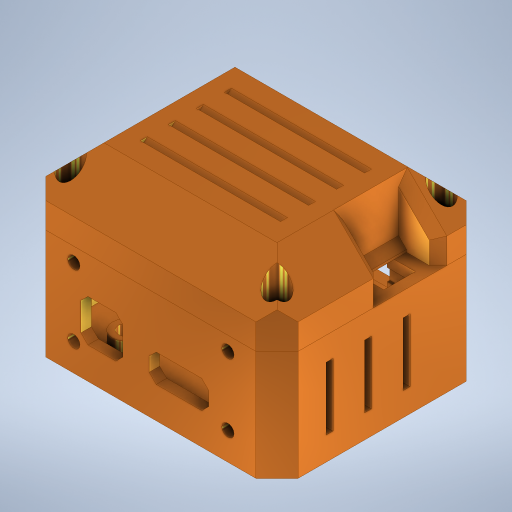
# Autodesk Inventor part: ModuloIndBase
Saved by Autodesk Inventor 2024.2 (Build 282272000, 272)
## iProperties
Created: 2024-09-07
Part Number: ModuloIndBase
Material: Generic
Document SubType Name: Modeling
Designer: Admin
Density: 1 g/cm^3
Appearance: Metal 1600F Hot
Author: Admin
Autodesk Inventor part; units mm, degrees
ref_plane "YZ Plane" through (0, 0, 0) normal (1, 0, 0) x (0, 1, 0)
ref_plane "XZ Plane" through (0, 0, 0) normal (0, 1, 0) x (-1, 0, 0)
ref_plane "XY Plane" through (0, 0, 0) normal (0, 0, 1) x (1, 0, 0)
sketch "Sketch1" plane through (0, 0, 0) normal (0, 1, 0) x (-1, 0, 0)
  line L0 (30, 36) -> (-30, 36)
  line L1 (-30, 36) -> (-30, -36)
  line L2 (-30, -36) -> (30, -36)
  line L3 (30, -36) -> (30, 36)
  line L4 (30, 36) -> (-30, -36) construction
  line L5 (-30, 36) -> (30, -36) construction
  point P0 (0, 0)
  dimension "d0" = 72
  dimension "d1" = 60
  constraints: 12 end point, 2 midpoint, 2 parallel, 1 horizontal, 1 perpendicular
  measures "d0" distance of L2.end L0.start
  measures "d1" distance of L0.start L0.end
extrude "BaseBlock" add sketch "Sketch1" along normal blind 50
chamfer "ExteriorDetail" distance 6 angle 45 4 edges at (-30, 25, 36) (30, 25, 36) (30, 25, -36) (-30, 25, -36)
chamfer "ExteriorShell" distance 11.3 angle 45 4 edges at (-30, 0, 0) (0, 0, 36) (30, 0, 0) (0, 0, -36)
shell "Shell1" thickness 3 removed faces 1 at (10, 50, -10)
ref_plane "Work Plane1" through (0, 18.6, 0) normal (0, 1, 0) x (1, 0, 0)
split body "Split1" result two bodies by plane through (0, 18.6, 0) normal (0, 1, 0) first body at (29.5, 29.0667, 10)
sketch "Sketch2" plane through (0, 50, 0) normal (0, 1, 0) x (1, 0, 0)
  line L0 (30, -30) -> (30, 30) projected
  line L1 (24, 36) -> (30, 30) projected
  line L2 (-27, 28.7574) -> (-22.7574, 33) projected
  line L3 (-22.7574, 33) -> (22.7574, 33) projected
  line L4 (22.7574, 33) -> (27, 28.7574) projected
  line L5 (27, 28.7574) -> (27, -28.7574) projected
  line L6 (27, -28.7574) -> (22.7574, -33) projected
  line L7 (22.7574, -33) -> (-22.7574, -33) projected
  line L8 (-22.7574, -33) -> (-27, -28.7574) projected
  line L9 (-27, -28.7574) -> (-27, 28.7574) projected
  line L10 (-30, 30) -> (-24, 36) projected
  line L11 (-30, 30) -> (-30, -30) projected
  line L12 (-24, -36) -> (-30, -30) projected
  line L13 (-24, -36) -> (24, -36) projected
  line L14 (30, -30) -> (24, -36) projected
  line L15 (30, -30) -> (30, 30) projected
  line L16 (24, 36) -> (30, 30) projected
  line L17 (24, 36) -> (-24, 36) projected
  point P0 (0, 0)
extrude "Extrusion2" add sketch "Sketch2" against normal blind 3 contours L14 L13 L12 L11 L10 L17 L1 L0 | L2 L3 L4 L5 L6 L7 L8 L9 bodies 2
sketch "Sketch4" plane through (-24, 18.6, -36) normal (0, -1, 0) x (1, 0, 0)
  line L0 (46.7574, 69) -> (51, 64.7574) projected
  line L1 (48.8787, 66.8787) -> (47.4645, 65.4645)
  line L2 (48.8787, 66.8787) -> (50.8787, 66.8787) construction
  circle A0 centre (47.4645, 65.4645) radius 2.25
  circle A1 centre (47.4645, 65.4645) radius 4
  line L3 (51, 64.7574) -> (51, 7.2426) projected
  line L4 (51, 36) -> (-3, 36) construction
  line L5 (-3, 7.2426) -> (-3, 64.7574) projected
  line L6 (51, 36) -> (105, 36) construction
  line L7 (24, 36) -> (24, 26) construction
  circle A2 centre (47.4645, 6.5355) radius 2.25
  circle A3 centre (47.4645, 6.5355) radius 4
  circle A4 centre (0.5355, 65.4645) radius 2.25
  circle A5 centre (0.5355, 65.4645) radius 4
  circle A6 centre (0.5355, 6.5355) radius 2.25
  circle A7 centre (0.5355, 6.5355) radius 4
  point P0 (48.1498, 67.6075)
  point P1 (49.6075, 66.1498)
  dimension "d23" = 2
  dimension "d24" = 135
  dimension "d25" = 4.5
  dimension "d27" = 8
  constraints: 10 end point, 8 centre point, 6 symmetric about line, 5 coincident, 4 midpoint, 2 equal length, 2 horizontal, 1 perpendicular, 1 vertical, 6 other
  measures "d23" distance of L1.start L1.end
  measures "d24" angle of L1 L2
  measures "d25" diameter of A0
  measures "d27" diameter of A1
extrude "Extrusion3" add sketch "Sketch4" against normal through all bodies 2
extrude "Extrusion4" cut sketch "Sketch4" against normal through all contours A0 L0 | L0 A0 | A2 | A4 | A6 bodies 2
sketch "Sketch5" plane through (0, 47, 0) normal (0, -1, 0) x (1, 0, 0)
  line L0 (0, 0) -> (1, 0) construction
  line L1 (-18, -19) -> (20, -19) construction
  line L2 (20, -19) -> (20, 19) construction
  line L3 (20, 19) -> (-18, 19) construction
  line L4 (-18, 19) -> (-18, -19) construction
  line L5 (-18, -19) -> (20, 19) construction
  line L6 (20, -19) -> (-18, 19) construction
  circle A0 centre (-18, -19) radius 1.6
  line L7 (-30, 30) -> (-30, -30) projected
  circle A1 centre (-18, -19) radius 4
  circle A2 centre (-18, -19) radius 2.275
  circle A3 centre (20, -19) radius 4
  circle A4 centre (20, -19) radius 2.275
  circle A5 centre (20, -19) radius 1.6
  circle A6 centre (20, 19) radius 4
  circle A7 centre (20, 19) radius 2.275
  circle A8 centre (20, 19) radius 1.6
  circle A9 centre (-18, 19) radius 4
  circle A10 centre (-18, 19) radius 2.275
  circle A11 centre (-18, 19) radius 1.6
  circle A12 centre (20, 19) radius 3.5
  dimension "d35" = 38
  dimension "d36" = 38
  dimension "d38" = 12
  dimension "d39" = 3.2
  dimension "d40" = 8
  dimension "d41" = 4.55
  dimension "d44" = 360
  dimension "d50" = 7
  constraints: 14 end point, 13 centre point, 7 coincident, 2 horizontal, 2 midpoint, 2 parallel, 1 perpendicular, 25 other
  measures "d35" distance of L3.end L2.end
  measures "d36" distance of L2.end L1.end
  measures "d38" distance between parallel lines of L4 L7
  measures "d39" diameter of A0
  measures "d40" diameter of A1
  measures "d41" diameter of A2
  measures "d50" diameter of A12
extrude "Extrusion5" cut sketch "Sketch5" against normal blind 3.2 contours A0 | A5 | A7 | A8 | A11 bodies 2
extrude "Extrusion6" add sketch "Sketch5" along normal blind 3.2 contours A1 | A3 | A9 bodies 2
extrude "Extrusion7" add sketch "Sketch5" along normal blind 3.2 contours A12 bodies 2
sketch "Sketch6" plane through (-21.5936, 47, -33) normal (0, 0, 1) x (1, 0, 0)
  line L0 (43.1873, 0) -> (0, 0) projected
  line L1 (-2.4064, -28.4) -> (45.5936, -28.4) projected
  line L2 (29.5936, 0) -> (21.5936, 0)
  line L3 (21.5936, 0) -> (21.5936, -28.4)
  line L4 (21.5936, -28.4) -> (29.5936, -28.4)
  line L5 (29.5936, -28.4) -> (29.5936, 0)
  line L6 (-8.4064, -28.4) -> (-8.4064, 3) projected
  line L7 (29.5936, -28.4) -> (25.0936, -28.4)
  line L8 (25.0936, -28.4) -> (25.0936, -25.4)
  line L9 (25.0936, -25.4) -> (29.5936, -25.4)
  line L10 (29.5936, -25.4) -> (29.5936, -28.4)
  line L11 (29.5936, -25.4) -> (24.3936, -25.4)
  line L12 (24.3936, -25.4) -> (24.3936, -21.9)
  line L13 (24.3936, -21.9) -> (29.5936, -21.9)
  line L14 (29.5936, -21.9) -> (29.5936, -25.4)
  line L15 (29.5936, -21.9) -> (25.0936, -21.9)
  line L16 (25.0936, -21.9) -> (25.0936, -18.9)
  line L17 (25.0936, -18.9) -> (29.5936, -18.9)
  line L18 (29.5936, -18.9) -> (29.5936, -21.9)
  line L19 (29.5936, -18.9) -> (23.5936, -18.9)
  line L20 (23.5936, -18.9) -> (23.5936, 0)
  line L21 (23.5936, 0) -> (29.5936, 0)
  line L22 (29.5936, 0) -> (29.5936, -18.9)
  line L23 (29.5936, 0) -> (37.5936, 0)
  line L24 (37.5936, 0) -> (37.5936, -28.4)
  line L25 (37.5936, -28.4) -> (29.5936, -28.4)
  line L26 (29.5936, -28.4) -> (34.0936, -28.4)
  line L27 (34.0936, -28.4) -> (34.0936, -25.4)
  line L28 (34.0936, -25.4) -> (29.5936, -25.4)
  line L29 (29.5936, -25.4) -> (34.7936, -25.4)
  line L30 (34.7936, -25.4) -> (34.7936, -21.9)
  line L31 (34.7936, -21.9) -> (29.5936, -21.9)
  line L32 (29.5936, -21.9) -> (34.0936, -21.9)
  line L33 (34.0936, -21.9) -> (34.0936, -18.9)
  line L34 (34.0936, -18.9) -> (29.5936, -18.9)
  line L35 (29.5936, -18.9) -> (35.5936, -18.9)
  line L36 (35.5936, -18.9) -> (35.5936, 0)
  line L37 (35.5936, 0) -> (29.5936, 0)
  point P0 (21.5936, -47)
  point P1 (25.0936, -21.9)
  point P2 (23.5936, 0)
  point P3 (21.5936, 0)
  point P4 (34.0936, -28.4)
  point P5 (37.5936, -28.4)
  point P6 (37.5936, 0)
  point P7 (35.5936, 0)
  point P8 (34.0936, -21.9)
  dimension "d53" = 30
  dimension "d54" = 8
  dimension "d55" = 4.5
  dimension "d56" = 3
  dimension "d57" = 3.5
  dimension "d58" = 5.2
  dimension "d59" = 3
  dimension "d60" = 4.5
  dimension "d61" = 2
  constraints: 70 end point, 10 parallel, 10 symmetric about line, 5 horizontal, 5 perpendicular, 3 point on line, 1 midpoint
  measures "d53" distance between parallel lines of L6 L3
  measures "d54" distance between parallel lines of L3 L5
  measures "d55" distance of L8.end L9.end
  measures "d56" distance of L7.end L8.end
  measures "d57" distance of L11.end L12.end
  measures "d58" distance of L12.end L13.end
  measures "d59" distance of L15.end L16.end
  measures "d60" distance of L16.end L17.end
  measures "d61" distance between parallel lines of L3 L20
extrude "Extrusion8" add sketch "Sketch6" along normal blind 8 contours L24 L1 L27 L29 L30 L31 L33 L35 L36 L0 | L20 L19 L16 L13 L12 L11 L8 L1 L3 L0 bodies 2
mirror "Mirror1" about plane through (0, 0, 0) normal (0, 0, 1) of "Extrusion8" bodies 2
sketch "Sketch7" plane through (30, 50, 30) normal (1, 0, 0) x (0, 0, -1)
  line L0 (46.5, -9) -> (29.5, -9)
  line L1 (29.5, -9) -> (29.5, -17)
  line L2 (29.5, -17) -> (46.5, -17)
  line L3 (46.5, -17) -> (46.5, -9)
  line L4 (66, -31.4) -> (66, 0) projected
  line L5 (0, 0) -> (60, 0) projected
  line L6 (22, -21) -> (10, -21)
  line L7 (10, -21) -> (10, -9)
  line L8 (10, -9) -> (22, -9)
  line L9 (22, -9) -> (22, -21)
  line L10 (60, -31.4) -> (0, -31.4) projected
  line L11 (-6, 0) -> (-6, -31.4) projected
  point P0 (30, -50)
  dimension "d72" = 17
  dimension "d73" = 8
  dimension "d74" = 19.5
  dimension "d75" = 9
  dimension "d77" = 16
  dimension "d78" = 12
  dimension "d79" = 12
  dimension "d80" = 9
  constraints: 16 end point, 4 parallel, 2 horizontal, 2 perpendicular
  measures "d72" distance of L1.end L2.end
  measures "d73" distance of L2.end L0.start
  measures "d74" distance between parallel lines of L4 L3
  measures "d75" distance between parallel lines of L5 L0
  measures "d77" distance between parallel lines of L11 L7
  measures "d78" distance of L7.end L8.end
  measures "d79" distance of L8.end L6.start
  measures "d80" distance between parallel lines of L5 L8
extrude "Extrusion9" cut sketch "Sketch7" against normal blind 3 bodies 2
mirror "Mirror2" about plane through (0, 0, 0) normal (1, 0, 0) of "Extrusion9" bodies 2
chamfer "Chamfer3" distance 2 angle 45 16 edges at (28.5, 33, -16.5) (28.5, 41, -16.5) (28.5, 41, 0.5) (28.5, 33, 0.5) (28.5, 29, 8) (28.5, 41, 8) (28.5, 41, 20) (28.5, 29, 20) (-28.5, 41, 20) (-28.5, 41, 0.5) (-28.5, 41, 8) (-28.5, 41, -16.5) (-28.5, 33, -16.5) (-28.5, 29, 8) (-28.5, 33, 0.5) (-28.5, 29, 20)
sketch "Sketch9" plane through (30, 50, 30) normal (1, 0, 0) x (0, 0, -1)
  line L0 (60, 0) -> (60, -31.4) construction
  line L1 (60, -31.4) -> (60, -27.4) construction
  line L2 (60, -27.4) -> (52, -27.4) construction
  circle A0 centre (52, -27.4) radius 1.75
  line L3 (2.4064, -31.4) -> (57.5936, -31.4) projected
  line L4 (30, -31.4) -> (30, 0) construction
  line L5 (2.4064, -3) -> (57.5936, -3) projected
  circle A1 centre (8, -27.4) radius 1.75
  circle A2 centre (52, -7.9) radius 1.75
  circle A3 centre (8, -7.9) radius 1.75
  point P0 (30, -50)
  dimension "d87" = 4
  dimension "d88" = 3.5
  dimension "d89" = 8
  dimension "d97" = 19.5
  constraints: 6 end point, 4 centre point, 2 perpendicular, 1 coincident, 1 midpoint, 1 point on line, 1 symmetric about line, 1 vertical, 5 other
  measures "d87" distance of L0.end L1.end
  measures "d88" diameter of A0
  measures "d89" distance of L1.end L2.end
  measures "d97" distance of A0.centre A2.centre
extrude "Extrusion10" cut sketch "Sketch9" against normal blind 3 bodies 2
mirror "Mirror3" about plane through (0, 0, 0) normal (1, 0, 0) of "Extrusion10" bodies 2
sketch "Sketch11" plane through (-24, 50, 36) normal (0, 0, 1) x (1, 0, 0)
  line L0 (10, -24.7) -> (9, -24.7)
  line L1 (9, -24.7) -> (9, -6.7)
  line L2 (9, -6.7) -> (10, -6.7)
  line L3 (10, -6.7) -> (10, -24.7)
  line L4 (48, -31.4) -> (0, -31.4) projected
  line L5 (-6, 0) -> (-6, -31.4) projected
  point P0 (24, -50)
  point P1 (9, -15.7)
  dimension "d108" = 1
  dimension "d109" = 18
  dimension "d110" = 15.7
  dimension "d111" = 15
  constraints: 8 end point, 2 parallel, 1 horizontal, 1 midpoint, 1 perpendicular
  measures "d108" distance of L1.end L2.end
  measures "d109" distance of L0.end L1.end
  measures "d110" distance from line of L4 point (9, -15.7)
  measures "d111" distance between parallel lines of L5 L1
extrude "Extrusion12" cut sketch "Sketch11" against normal through all bodies 2
chamfer "Chamfer4" distance 1 angle 45 4 edges at (-15, 34.3, 36) (-15, 34.3, -36) (-14, 34.3, -33) (-14, 34.3, 33)
pattern_linear "Rectangular Pattern1" count 3 spacing 11 along (1, 0, 0) of "Extrusion12", "Chamfer4" bodies 2
sketch "Sketch14" plane through (-24, 18.6, 36) normal (0, 1, 0) x (1, 0, 0)
  line L0 (51, 3) -> (47.4645, 6.5355) construction
  circle A0 centre (47.4645, 6.5355) radius 4
  circle A1 centre (47.4645, 6.5355) radius 1.6
  line L1 (24, 36) -> (29, 36) construction
  line L2 (24, 36) -> (24, 31) construction
  line L3 (46.7574, 3) -> (51, 7.2426) projected
  circle A2 centre (47.4645, 65.4645) radius 4
  circle A3 centre (47.4645, 65.4645) radius 1.6
  circle A4 centre (0.5355, 6.5355) radius 4
  circle A5 centre (0.5355, 6.5355) radius 1.6
  circle A6 centre (0.5355, 65.4645) radius 4
  circle A7 centre (0.5355, 65.4645) radius 1.6
  dimension "d131" = 8
  dimension "d135" = 90
  constraints: 8 centre point, 6 end point, 6 symmetric about line, 2 coincident, 1 horizontal, 1 vertical, 6 other
  measures "d131" diameter of A0
  measures "d135" angle of L3 L0
extrude "Extrusion14" add sketch "Sketch14" against normal through all bodies 3
sketch "Sketch13" plane through (0, 0, 0) normal (0, -1, 0) x (1, 0, 0)
  line L0 (-27, 33) -> (-23.4645, 29.4645) construction
  line L1 (-27, 33) -> (-22, 33) construction
  circle A0 centre (-23.4645, 29.4645) radius 1.6
  circle A1 centre (-23.4645, 29.4645) radius 3.25
  line L2 (0, 0) -> (-5, 0) construction
  line L3 (0, 0) -> (0, 5) construction
  circle A2 centre (23.4645, 29.4645) radius 1.6
  circle A3 centre (23.4645, 29.4645) radius 3.25
  line L4 (-24, -36) -> (-27, -33)
  line L5 (-27, -33) -> (-23.4645, -29.4645) construction
  line L6 (-27, -33) -> (-22, -33) construction
  circle A4 centre (-23.4645, -29.4645) radius 1.6
  circle A5 centre (-23.4645, -29.4645) radius 3.25
  line L7 (24, -36) -> (-24, -36)
  circle A6 centre (23.4645, -29.4645) radius 1.6
  circle A7 centre (23.4645, -29.4645) radius 3.25
  point P0 (-24, 36)
  point P1 (24, 36)
  dimension "d120" = 5
  dimension "d121" = 45
  dimension "d122" = 3.2
  dimension "d123" = 6.5
  constraints: 16 end point, 11 symmetric about line, 8 centre point, 6 coincident, 2 horizontal, 1 equal length, 1 vertical, 6 other
  measures "d120" distance of L0.start L0.end
  measures "d121" angle of L0 L1
  measures "d122" diameter of A0
  measures "d123" diameter of A1
extrude "Extrusion13" cut sketch "Sketch13" against normal blind 14 contours A0 | A1 | A2 | A3 | A4 | A5 | A6 | A7 bodies 3
sketch "Sketch15" plane through (-24, 18.6, 36) normal (0, 1, 0) x (1, 0, 0)
  line L0 (24, 69) -> (24, 60.7)
  line L1 (24, 60.7) -> (40, 60.7)
  line L2 (40, 60.7) -> (40, 68.7)
  line L3 (54, 66) -> (54, 6) projected
  line L4 (43, 57.7) -> (21, 57.7)
  line L5 (21, 57.7) -> (21, 72)
  line L6 (21, 72) -> (43, 72)
  line L7 (43, 72) -> (43, 57.7)
  line L8 (24, 36) -> (34, 36) construction
  line L9 (40, 60.7) -> (40, 72)
  line L10 (24, 60.7) -> (24, 72)
  line L11 (24, 3) -> (24, 11.3)
  line L12 (24, 11.3) -> (40, 11.3)
  line L13 (40, 11.3) -> (40, 3.3)
  line L14 (43, 14.3) -> (21, 14.3)
  line L15 (21, 14.3) -> (21, 0)
  line L16 (21, 0) -> (43, 0)
  line L17 (43, 0) -> (43, 14.3)
  line L18 (40, 11.3) -> (40, 0)
  line L19 (24, 11.3) -> (24, 0)
  line L20 (0, 72) -> (48, 72) projected
  point P0 (24, 69)
  dimension "d138" = 8
  dimension "d139" = 16
  dimension "d140" = 14
  dimension "d141" = 3
  dimension "d150" = 11.3
  dimension "d151" = 0
  constraints: 38 end point, 10 symmetric about line, 6 point on line, 3 parallel, 2 perpendicular, 1 horizontal, 1 other
  measures "d138" distance of L1.end L2.end
  measures "d139" distance of L0.end L1.end
  measures "d140" distance between parallel lines of L3 L2
  measures "d141" distance between parallel lines of L1 L4
  measures "d150" distance between parallel lines of L6 L1
  measures "d151" distance between parallel lines of L6 L20
extrude "Extrusion15" add sketch "Sketch15" against normal through all contours L0 L1 L2 L9 L6 L7 L4 L5 L10 | L19 L16 L15 L14 L17 L18 L13 L12 L11 bodies 3
extrude "Extrusion16" cut sketch "Sketch15" against normal through all contours L10 L6 L9 L2 L1 L0 | L11 L12 L13 L18 L16 L19 bodies 3
chamfer "Chamfer5" distance 2.5 angle 45 8 edges at (0, 5.65, -30.35) (0, 14.95, -36) (16, 5.65, -30.35) (16, 14.95, -36) (0, 5.65, 30.35) (0, 14.95, 36) (16, 14.95, 36) (16, 5.65, 30.35)
sketch "Sketch17" plane through (0, 0, 0) normal (0, 0, 1) x (1, 0, 0)
  line L0 (0, 0) -> (-11, 0) construction
  line L1 (-11, 0) -> (-13, 0)
  line L2 (-13, 0) -> (-16.5753, 3)
  line L3 (-16.5753, 3) -> (-14.5753, 3)
  line L4 (-14.5753, 3) -> (-11, 0)
  line L5 (-5, 0) -> (-8.5753, 3)
  line L6 (-8.5753, 3) -> (-6.5753, 3)
  line L7 (-6.5753, 3) -> (-3, 0)
  line L8 (-3, 0) -> (-5, 0)
  line L9 (3, 0) -> (-0.5753, 3)
  line L10 (-0.5753, 3) -> (1.4247, 3)
  line L11 (1.4247, 3) -> (5, 0)
  line L12 (5, 0) -> (3, 0)
  line L13 (11, 0) -> (7.4247, 3)
  line L14 (7.4247, 3) -> (9.4247, 3)
  line L15 (9.4247, 3) -> (13, 0)
  line L16 (13, 0) -> (11, 0)
  dimension "d152" = 11
  dimension "d153" = 2
  dimension "d154" = 2
  dimension "d157" = 40
  dimension "d160" = 8
  constraints: 34 end point, 1 horizontal, 1 parallel, 24 other
  measures "d152" distance of L0.start L0.end
  measures "d153" distance of L0.end L1.end
  measures "d154" distance of L2.end L3.end
  measures "d157" angle of L1 L4
  measures "d160" distance of L1.end L5.start
extrude "Extrusion17" cut sketch "Sketch17" along normal mid plane 40 bodies 3
sketch "Sketch18" plane through (0, 18.6, 24.7) normal (0, 0, 1) x (1, 0, 0)
  line L0 (0, 0) -> (16, 0) projected
  line L1 (0, 0) -> (0, -15.0645) projected
  line L2 (16, 0) -> (0, 0)
  line L3 (0, 0) -> (0, -3)
  line L4 (0, -3) -> (16, -3)
  line L5 (16, -3) -> (16, 0)
  point P0 (0, -18.6)
  dimension "d167" = 3
  constraints: 8 end point, 2 parallel, 1 horizontal, 1 perpendicular, 1 point on line
  measures "d167" distance of L3.end L2.end
extrude "Extrusion18" add sketch "Sketch18" along normal blind 2.3 bodies 3
chamfer "Chamfer6" distance 2.3 angle 45 1 edges at (8, 15.6, 27)
mirror "Mirror4" about plane through (0, 0, 0) normal (0, 0, 1) of "Extrusion18", "Chamfer6" bodies 3
